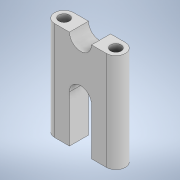
# Autodesk Inventor part: suction_clip_2_bottom
Saved by Autodesk Inventor 2022 (Build 260153000, 153)
## iProperties
Created: 2022-09-13
Part Number: suction_clip_2_bottom
Material: Generic
Document SubType Name: Modeling
Designer: dsdan
Density: 1 g/cm^3
Appearance: Default
Author: dsdan
Autodesk Inventor part; units mm, degrees
ref_plane "YZ Plane" through (0, 0, 0) normal (1, 0, 0) x (0, 1, 0)
ref_plane "XZ Plane" through (0, 0, 0) normal (0, 1, 0) x (-1, 0, 0)
ref_plane "XY Plane" through (0, 0, 0) normal (0, 0, 1) x (1, 0, 0)
sketch "Sketch1" plane through (0, 0, 0) normal (0, 1, 0) x (-1, 0, 0)
  circle A0 centre (0, 0) radius 1.55
  circle A1 centre (-15, 0) radius 1.55
  line L0 (0, 0) -> (-15, 0) construction
  line L1 (0, 2.75) -> (-15, 2.75)
  line L2 (-15, -2.75) -> (0, -2.75)
  arc A2 (0, -2.75) -> (0, 2.75) centre (0, 0) ccw
  arc A3 (-15, 2.75) -> (-15, -2.75) centre (-15, 0) ccw
  point P0 (-7.5, 0)
  dimension "d0" = 3.1
  dimension "d1" = 15
  dimension "d2" = 20.5
  constraints: 8 end point, 4 centre point, 4 point on circle, 4 tangent, 1 coincident, 1 equal radius, 1 horizontal, 1 midpoint, 1 parallel
  measures "d0" diameter of A0
  measures "d1" distance of L0.end L0.start
extrude "Extrusion1" add sketch "Sketch1" along normal blind 28.6
sketch "Sketch2" plane through (0, 0, 2.75) normal (0, 0, 1) x (1, 0, 0)
  line L0 (15, 28.6) -> (0, 28.6) projected
  circle A0 centre (7.5, 28.6) radius 3.2
  line L1 (7.5, 13.6) -> (7.5, -5.0521) construction
  line L2 (4.3, 13.6) -> (4.3, -5.0521)
  line L3 (10.7, -5.0521) -> (10.7, 13.6)
  arc A1 (10.7, 13.6) -> (4.3, 13.6) centre (7.5, 13.6) ccw
  arc A2 (4.3, -5.0521) -> (10.7, -5.0521) centre (7.5, -5.0521) ccw
  line L4 (0, 28.6) -> (15, 28.6) projected
  point P0 (0, 0)
  point P1 (4.3, 28.6)
  point P2 (10.7, 28.6)
  point P3 (7.5, 4.274)
  dimension "d5" = 6.4
  dimension "d8" = 15
  constraints: 8 end point, 4 point on circle, 4 tangent, 3 centre point, 3 midpoint, 1 equal radius, 1 parallel, 1 point on line, 1 vertical
  measures "d5" diameter of A0
  measures "d8" distance of A0.centre L1.start
extrude "Extrusion2" cut sketch "Sketch2" against normal through all contours A0 L0 | A1 L3 A2 L2 picked at (6.7016, 27.3821)
body "Solid1"
